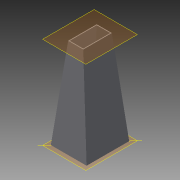
# Autodesk Inventor part: NewHorn
Saved by Autodesk Inventor 2015 (Build 190159000, 159)
## iProperties
Created: 2014-03-24
Part Number: NewHorn
Material: Generic
Document SubType Name: Modeling
Designer: jad211
Density: 1 g/cm^3
Appearance: Default
Author: jad211
Autodesk Inventor part; units mm, degrees
ref_plane "YZ Plane" through (0, 0, 0) normal (1, 0, 0) x (0, 1, 0)
ref_plane "XZ Plane" through (0, 0, 0) normal (0, 1, 0) x (-1, 0, 0)
ref_plane "XY Plane" through (0, 0, 0) normal (0, 0, 1) x (1, 0, 0)
sketch "Sketch1" plane through (0, 0, 0) normal (0, 0, 1) x (1, 0, 0)
  line L0 (-10.5, -12.5) -> (10.5, -12.5)
  line L1 (10.5, -12.5) -> (10.5, 12.5)
  line L2 (10.5, 12.5) -> (-10.5, 12.5)
  line L3 (-10.5, 12.5) -> (-10.5, -12.5)
  line L4 (-10.5, -12.5) -> (10.5, 12.5) construction
  line L5 (10.5, -12.5) -> (-10.5, 12.5) construction
  point P0 (0, 0)
  dimension "d0" = 21
  dimension "d1" = 25
  constraints: 12 end point, 2 midpoint, 2 parallel, 1 horizontal, 1 perpendicular
  measures "d0" distance of L2.end L1.end
  measures "d1" distance of L1.end L0.end
ref_plane "Work Plane2" through (10.5, -12.5, 54) normal (0, 0, 1) x (0, 1, 0)
ref_plane "Work Plane1" through (10.5, -12.5, 0) normal (0, 0, 1) x (0, 1, 0)
sketch "Sketch2" plane through (10.5, -12.5, 54) normal (0, 0, 1) x (0, 1, 0)
  line L0 (4.1005, 6.0505) -> (20.8995, 6.0505)
  line L1 (20.8995, 6.0505) -> (20.8995, 14.9495)
  line L2 (20.8995, 14.9495) -> (4.1005, 14.9495)
  line L3 (4.1005, 14.9495) -> (4.1005, 6.0505)
  line L4 (4.1005, 6.0505) -> (20.8995, 14.9495) construction
  line L5 (20.8995, 6.0505) -> (4.1005, 14.9495) construction
  point P0 (12.5, 10.5)
  dimension "d3" = 16.799
  dimension "d4" = 8.899
  constraints: 12 end point, 2 midpoint, 2 parallel, 1 horizontal, 1 perpendicular
  measures "d3" distance of L2.end L1.end
  measures "d4" distance of L1.end L0.end
loft "Loft1" add profiles "Sketch2", "Sketch1"
sketch "Sketch4" plane through (10.5, -12.5, 0) normal (0, 0, -1) x (-1, 0, 0)
  line L0 (0.5, 0.5) -> (20.5, 0.5)
  line L1 (20.5, 0.5) -> (20.5, 24.5)
  line L2 (20.5, 24.5) -> (0.5, 24.5)
  line L3 (0.5, 24.5) -> (0.5, 0.5)
  line L4 (0.5, 0.5) -> (20.5, 24.5) construction
  line L5 (20.5, 0.5) -> (0.5, 24.5) construction
  point P0 (10.5, 12.5)
  dimension "d9" = 20
  dimension "d10" = 24
  constraints: 12 end point, 2 midpoint, 2 parallel, 1 horizontal, 1 perpendicular
  measures "d9" distance of L2.end L1.end
  measures "d10" distance of L1.end L0.end
sketch "Sketch5" plane through (-4.4495, 8.3995, 54) normal (0, 0, 1) x (1, 0, 0)
  line L0 (0.5, -16.299) -> (8.399, -16.299)
  line L1 (8.399, -16.299) -> (8.399, -0.5)
  line L2 (8.399, -0.5) -> (0.5, -0.5)
  line L3 (0.5, -0.5) -> (0.5, -16.299)
  line L4 (0.5, -16.299) -> (8.399, -0.5) construction
  line L5 (8.399, -16.299) -> (0.5, -0.5) construction
  point P0 (4.4495, -8.3995)
  dimension "d11" = 7.899
  dimension "d12" = 15.799
  constraints: 12 end point, 2 midpoint, 2 parallel, 1 horizontal, 1 perpendicular
  measures "d11" distance of L2.end L1.end
  measures "d12" distance of L1.end L0.end
loft "Loft2" cut profiles "Sketch5", "Sketch4"
body "Solid1"
